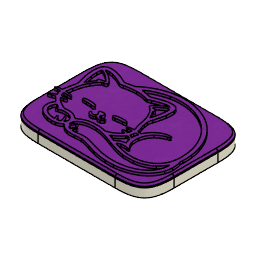
Sleeping Cat (Autodesk Fusion 360 design; units mm, degrees)
Autodesk Fusion 360 part; units mm, degrees
sketch "Imported SVG" plane through (0, 0, 0) normal (0, 0, 1) x (1, 0, 0)
  spline S0 degree 3 poles (44.1719, -83.1207) (37.6327, -82.7636) (28.995, -81.3586) (21.6671, -79.4603) knots 0 0 0 0 1 1 1 1
  spline S1 degree 3 poles (21.6671, -79.4603) (19.4843, -78.8948) (14.067, -77.2897) (9.6286, -75.8934) knots 0 0 0 0 1 1 1 1
  spline S2 degree 3 poles (9.6286, -75.8934) (0.5567, -73.0394) (-2.952, -72.1681) (-6.8676, -71.7971) knots 0 0 0 0 1 1 1 1
  spline S3 degree 3 poles (-6.8676, -71.7971) (-9.7124, -71.5276) (-14.5477, -71.7698) (-18.1526, -72.3625) knots 0 0 0 0 1 1 1 1
  spline S4 degree 3 poles (-18.1526, -72.3625) (-21.044, -72.8379) (-28.1463, -72.7506) (-30.562, -72.2099) knots 0 0 0 0 1 1 1 1
  spline S5 degree 3 poles (-30.562, -72.2099) (-33.3375, -71.5887) (-35.9478, -70.638) (-37.6802, -69.6171) knots 0 0 0 0 1 1 1 1
  spline S6 degree 3 poles (-37.6802, -69.6171) (-39.1993, -68.722) (-42.056, -66.0985) (-42.8145, -64.902) knots 0 0 0 0 1 1 1 1
  spline S7 degree 3 poles (-42.8145, -64.902) (-43.2338, -64.2406) (-43.2338, -64.2406) (-43.9885, -64.9292) knots 0 0 0 0 1 1 1 1
  spline S8 degree 3 poles (-43.9885, -64.9292) (-46.1715, -66.921) (-49.1149, -68.3543) (-53.2379, -69.4332) knots 0 0 0 0 1 1 1 1
  spline S9 degree 3 poles (-53.2379, -69.4332) (-55.2617, -69.9628) (-56.2025, -70.0467) (-59.9568, -70.0326) knots 0 0 0 0 1 1 1 1
  spline S10 degree 3 poles (-59.9568, -70.0326) (-63.7018, -70.0185) (-64.7913, -69.9128) (-67.6205, -69.2894) knots 0 0 0 0 1 1 1 1
  spline S11 degree 3 poles (-67.6205, -69.2894) (-75.9739, -67.4486) (-82.0673, -63.6492) (-85.307, -58.2616) knots 0 0 0 0 1 1 1 1
  spline S12 degree 3 poles (-85.307, -58.2616) (-85.6218, -57.738) (-86.2028, -56.4878) (-86.5979, -55.4834) knots 0 0 0 0 1 1 1 1
  spline S13 degree 3 poles (-86.5979, -55.4834) (-87.2545, -53.8147) (-87.3163, -53.3493) (-87.3142, -50.0854) knots 0 0 0 0 1 1 1 1
  spline S14 degree 3 poles (-87.3142, -50.0854) (-87.3121, -46.83) (-87.2471, -46.342) (-86.5803, -44.5775) knots 0 0 0 0 1 1 1 1
  spline S15 degree 3 poles (-86.5803, -44.5775) (-85.9476, -42.9035) (-84.7731, -40.6976) (-83.7154, -39.1965) knots 0 0 0 0 1 1 1 1
  spline S16 degree 3 poles (-83.7154, -39.1965) (-83.4549, -38.8267) (-83.6508, -38.5397) (-84.9772, -37.3485) knots 0 0 0 0 1 1 1 1
  spline S17 degree 3 poles (-84.9772, -37.3485) (-86.9937, -35.5374) (-88.0353, -34.4909) (-89.9901, -32.3117) knots 0 0 0 0 1 1 1 1
  spline S18 degree 3 poles (-89.9901, -32.3117) (-91.5745, -30.5454) (-91.5745, -30.5454) (-96.4559, -32.3963) knots 0 0 0 0 1 1 1 1
  spline S19 degree 3 poles (-96.4559, -32.3963) (-100.5126, -33.9346) (-101.4401, -34.2004) (-101.946, -33.9699) knots 0 0 0 0 1 1 1 1
  spline S20 degree 3 poles (-101.946, -33.9699) (-102.6861, -33.6327) (-102.7356, -32.8037) (-102.0562, -32.1243) knots 0 0 0 0 1 1 1 1
  spline S21 degree 3 poles (-102.0562, -32.1243) (-101.3048, -31.373) (-98.7657, -29.9625) (-95.8079, -28.6533) knots 0 0 0 0 1 1 1 1
  spline S22 degree 3 poles (-95.8079, -28.6533) (-94.3526, -28.0093) (-93.1244, -27.4603) (-93.0784, -27.4334) knots 0 0 0 0 1 1 1 1
  spline S23 degree 3 poles (-93.0784, -27.4334) (-93.0324, -27.4064) (-93.3604, -26.525) (-93.8074, -25.4747) knots 0 0 0 0 1 1 1 1
  spline S24 degree 3 poles (-93.8074, -25.4747) (-94.6338, -23.5327) (-95.411, -20.6554) (-95.411, -19.5379) knots 0 0 0 0 1 1 1 1
  spline S25 degree 3 poles (-95.411, -19.5379) (-95.411, -19.1987) (-95.5598, -18.8682) (-95.7417, -18.8034) knots 0 0 0 0 1 1 1 1
  spline S26 degree 3 poles (-95.7417, -18.8034) (-95.9236, -18.7386) (-97.998, -18.7963) (-100.3516, -18.9316) knots 0 0 0 0 1 1 1 1
  spline S27 degree 3 poles (-100.3516, -18.9316) (-105.0411, -19.2011) (-106.0471, -19.02) (-106.2103, -17.8766) knots 0 0 0 0 1 1 1 1
  spline S28 degree 3 poles (-106.2103, -17.8766) (-106.3839, -16.6604) (-104.273, -15.967) (-98.7253, -15.4178) knots 0 0 0 0 1 1 1 1
  spline S29 degree 3 poles (-98.7253, -15.4178) (-97.1284, -15.2597) (-95.8104, -15.1073) (-95.7963, -15.0792) knots 0 0 0 0 1 1 1 1
  spline S30 degree 3 poles (-95.7963, -15.0792) (-95.7821, -15.0511) (-95.6257, -13.6589) (-95.4487, -11.9854) knots 0 0 0 0 1 1 1 1
  spline S31 degree 3 poles (-95.4487, -11.9854) (-95.2716, -10.3119) (-94.7182, -7.2163) (-94.2189, -5.1062) knots 0 0 0 0 1 1 1 1
  spline S32 degree 3 poles (-94.2189, -5.1062) (-93.7196, -2.9962) (-92.9464, 0.5526) (-92.5007, 2.7798) knots 0 0 0 0 1 1 1 1
  spline S33 degree 3 poles (-92.5007, 2.7798) (-91.5958, 7.3017) (-91.4237, 5.8765) (-94.0568, 15.6636) knots 0 0 0 0 1 1 1 1
  spline S34 degree 3 poles (-94.0568, 15.6636) (-94.4874, 17.2643) (-95.1952, 20.3599) (-95.6295, 22.5427) knots 0 0 0 0 1 1 1 1
  spline S35 degree 3 poles (-95.6295, 22.5427) (-97.4372, 31.6271) (-98.0013, 37.4542) (-97.5381, 42.2569) knots 0 0 0 0 1 1 1 1
  spline S36 degree 3 poles (-97.5381, 42.2569) (-96.6603, 51.359) (-94.0135, 55.105) (-87.5048, 56.4575) knots 0 0 0 0 1 1 1 1
  spline S37 degree 3 poles (-87.5048, 56.4575) (-81.1549, 57.7769) (-69.2652, 54.9101) (-57.1426, 49.1368) knots 0 0 0 0 1 1 1 1
  spline S38 degree 3 poles (-57.1426, 49.1368) (-53.1378, 47.2295) (-53.1378, 47.2295) (-48.2791, 48.4514) knots 0 0 0 0 1 1 1 1
  spline S39 degree 3 poles (-48.2791, 48.4514) (-45.6068, 49.1235) (-42.2762, 49.8288) (-40.8778, 50.0188) knots 0 0 0 0 1 1 1 1
  spline S40 degree 3 poles (-40.8778, 50.0188) (-38.3352, 50.3643) (-38.3352, 50.3643) (-36.1153, 52.2914) knots 0 0 0 0 1 1 1 1
  spline S41 degree 3 poles (-36.1153, 52.2914) (-29.682, 57.8762) (-22.2779, 62.5427) (-14.0516, 66.1972) knots 0 0 0 0 1 1 1 1
  spline S42 degree 3 poles (-14.0516, 66.1972) (-5.5262, 69.9846) (3.8871, 72.5528) (13.2439, 73.6442) knots 0 0 0 0 1 1 1 1
  spline S43 degree 3 poles (13.2439, 73.6442) (18.3627, 74.2413) (27.6961, 74.2377) (32.5805, 73.6368) knots 0 0 0 0 1 1 1 1
  spline S44 degree 3 poles (32.5805, 73.6368) (51.3464, 71.328) (68.3594, 63.9806) (81.7612, 52.397) knots 0 0 0 0 1 1 1 1
  spline S45 degree 3 poles (81.7612, 52.397) (93.211, 42.5006) (101.58, 29.8071) (106.4162, 15.0021) knots 0 0 0 0 1 1 1 1
  spline S46 degree 3 poles (106.4162, 15.0021) (108.8797, 7.4607) (109.4869, 4.8611) (110.4334, -2.1958) knots 0 0 0 0 1 1 1 1
  spline S47 degree 3 poles (110.4334, -2.1958) (111.1822, -7.7792) (111.3768, -13.2405) (110.9863, -17.7108) knots 0 0 0 0 1 1 1 1
  spline S48 degree 3 poles (110.9863, -17.7108) (110.6856, -21.1527) (110.6986, -21.4838) (111.1978, -23.0979) knots 0 0 0 0 1 1 1 1
  spline S49 degree 3 poles (111.1978, -23.0979) (112.7036, -27.9673) (113.1723, -31.5404) (113.0055, -36.8779) knots 0 0 0 0 1 1 1 1
  spline S50 degree 3 poles (113.0055, -36.8779) (112.8526, -41.772) (112.3877, -44.5762) (111.0572, -48.6302) knots 0 0 0 0 1 1 1 1
  spline S51 degree 3 poles (111.0572, -48.6302) (104.9608, -67.2056) (84.7258, -80.447) (58.7088, -82.8859) knots 0 0 0 0 1 1 1 1
  spline S52 degree 3 poles (58.7088, -82.8859) (54.8482, -83.2478) (48.4048, -83.3519) (44.1719, -83.1207) knots 0 0 0 0 1 1 1 1
  spline S53 degree 3 poles (59.6349, -76.2813) (73.1592, -74.7946) (83.8175, -70.8695) (92.7216, -64.0966) knots 0 0 0 0 1 1 1 1
  spline S54 degree 3 poles (92.7216, -64.0966) (95.3009, -62.1347) (99.2539, -57.9512) (100.9411, -55.3979) knots 0 0 0 0 1 1 1 1
  spline S55 degree 3 poles (100.9411, -55.3979) (104.5866, -49.8809) (106.8783, -42.5825) (106.68, -37.1208) knots 0 0 0 0 1 1 1 1
  spline S56 degree 3 poles (106.68, -37.1208) (106.5984, -34.8718) (106.5984, -34.8718) (105.5401, -36.8541) knots 0 0 0 0 1 1 1 1
  spline S57 degree 3 poles (105.5401, -36.8541) (103.3997, -40.8631) (99.8697, -45.3493) (96.5442, -48.2865) knots 0 0 0 0 1 1 1 1
  spline S58 degree 3 poles (96.5442, -48.2865) (89.2838, -54.6995) (80.4809, -58.4766) (69.1599, -60.0365) knots 0 0 0 0 1 1 1 1
  spline S59 degree 3 poles (69.1599, -60.0365) (64.995, -60.6103) (55.3281, -60.6926) (51.6974, -60.1851) knots 0 0 0 0 1 1 1 1
  spline S60 degree 3 poles (51.6974, -60.1851) (42.5072, -58.9004) (35.3971, -56.9631) (23.1224, -52.3992) knots 0 0 0 0 1 1 1 1
  spline S61 degree 3 poles (23.1224, -52.3992) (7.5582, -46.6122) (-1.8118, -44.1125) (-10.4797, -43.4351) knots 0 0 0 0 1 1 1 1
  spline S62 degree 3 poles (-10.4797, -43.4351) (-23.6948, -42.4023) (-35.2995, -46.4923) (-38.7857, -53.4116) knots 0 0 0 0 1 1 1 1
  spline S63 degree 3 poles (-38.7857, -53.4116) (-39.7884, -55.4016) (-39.8384, -60.4041) (-38.8556, -60.4041) knots 0 0 0 0 1 1 1 1
  spline S64 degree 3 poles (-38.8556, -60.4041) (-38.7388, -60.4041) (-38.2981, -59.6118) (-37.8762, -58.6433) knots 0 0 0 0 1 1 1 1
  spline S65 degree 3 poles (-37.8762, -58.6433) (-36.5382, -55.572) (-33.1377, -52.733) (-31.534, -53.3484) knots 0 0 0 0 1 1 1 1
  spline S66 degree 3 poles (-31.534, -53.3484) (-30.8188, -53.6229) (-31.0673, -54.2427) (-32.5652, -55.9214) knots 0 0 0 0 1 1 1 1
  spline S67 degree 3 poles (-32.5652, -55.9214) (-34.5051, -58.0955) (-35.4015, -60.035) (-35.5543, -62.3885) knots 0 0 0 0 1 1 1 1
  spline S68 degree 3 poles (-35.5543, -62.3885) (-35.6564, -63.9611) (-35.6002, -64.3037) (-35.1818, -64.6592) knots 0 0 0 0 1 1 1 1
  spline S69 degree 3 poles (-35.1818, -64.6592) (-34.6213, -65.1355) (-32.1243, -66.225) (-31.5933, -66.225) knots 0 0 0 0 1 1 1 1
  spline S70 degree 3 poles (-31.5933, -66.225) (-31.3998, -66.225) (-31.0343, -65.6418) (-30.7812, -64.9291) knots 0 0 0 0 1 1 1 1
  spline S71 degree 3 poles (-30.7812, -64.9291) (-29.807, -62.1862) (-27.3938, -59.6388) (-25.7511, -59.6192) knots 0 0 0 0 1 1 1 1
  spline S72 degree 3 poles (-25.7511, -59.6192) (-24.6173, -59.6056) (-24.6328, -60.2158) (-25.8056, -61.7648) knots 0 0 0 0 1 1 1 1
  spline S73 degree 3 poles (-25.8056, -61.7648) (-26.9421, -63.266) (-27.6777, -65.0368) (-27.6777, -66.2721) knots 0 0 0 0 1 1 1 1
  spline S74 degree 3 poles (-27.6777, -66.2721) (-27.6777, -66.9827) (-27.617, -67.02) (-26.4209, -67.0453) knots 0 0 0 0 1 1 1 1
  spline S75 degree 3 poles (-26.4209, -67.0453) (-24.3172, -67.0897) (-20.4251, -66.9827) (-20.2518, -66.8756) knots 0 0 0 0 1 1 1 1
  spline S76 degree 3 poles (-20.2518, -66.8756) (-20.1103, -66.7881) (-14.6329, -66.0458) (-10.5986, -65.5674) knots 0 0 0 0 1 1 1 1
  spline S77 degree 3 poles (-10.5986, -65.5674) (-8.5699, -65.3268) (-3.2912, -65.84) (-0.0019, -66.5975) knots 0 0 0 0 1 1 1 1
  spline S78 degree 3 poles (-0.0019, -66.5975) (3.1146, -67.3153) (5.2671, -67.9321) (15.1684, -70.9449) knots 0 0 0 0 1 1 1 1
  spline S79 degree 3 poles (15.1684, -70.9449) (26.3524, -74.3481) (32.8284, -75.6052) (44.5536, -76.6492) knots 0 0 0 0 1 1 1 1
  spline S80 degree 3 poles (44.5536, -76.6492) (46.5618, -76.828) (56.9717, -76.574) (59.6349, -76.2813) knots 0 0 0 0 1 1 1 1
  spline S81 degree 3 poles (-60.311, -63.2584) (-60.4008, -62.5) (-60.8841, -61.0559) (-61.3848, -60.0494) knots 0 0 0 0 1 1 1 1
  spline S82 degree 3 poles (-61.3848, -60.0494) (-62.347, -58.1155) (-62.3668, -57.4937) (-61.4662, -57.4937) knots 0 0 0 0 1 1 1 1
  spline S83 degree 3 poles (-61.4662, -57.4937) (-59.9519, -57.4937) (-57.7892, -60.1153) (-57.1235, -62.7578) knots 0 0 0 0 1 1 1 1
  spline S84 degree 3 poles (-57.1235, -62.7578) (-56.6476, -64.6472) (-56.6458, -64.6477) (-53.5746, -63.819) knots 0 0 0 0 1 1 1 1
  spline S85 degree 3 poles (-53.5746, -63.819) (-51.5221, -63.2652) (-51.5221, -63.2652) (-51.3465, -61.8599) knots 0 0 0 0 1 1 1 1
  spline S86 degree 3 poles (-51.3465, -61.8599) (-51.0498, -59.4857) (-51.7827, -57.1192) (-53.6657, -54.3703) knots 0 0 0 0 1 1 1 1
  spline S87 degree 3 poles (-53.6657, -54.3703) (-54.5053, -53.1447) (-54.4826, -52.4666) (-53.602, -52.4666) knots 0 0 0 0 1 1 1 1
  spline S88 degree 3 poles (-53.602, -52.4666) (-51.5314, -52.4666) (-48.4862, -56.3441) (-48.1335, -59.4298) knots 0 0 0 0 1 1 1 1
  spline S89 degree 3 poles (-48.1335, -59.4298) (-47.9172, -61.3222) (-47.8561, -61.3697) (-46.8691, -60.413) knots 0 0 0 0 1 1 1 1
  spline S90 degree 3 poles (-46.8691, -60.413) (-42.5188, -56.1965) (-45.7992, -49.1698) (-53.2099, -46.8305) knots 0 0 0 0 1 1 1 1
  spline S91 degree 3 poles (-53.2099, -46.8305) (-58.3274, -45.2152) (-65.3333, -45.7312) (-70.4631, -48.1013) knots 0 0 0 0 1 1 1 1
  spline S92 degree 3 poles (-70.4631, -48.1013) (-72.5845, -49.0814) (-73.4099, -49.2264) (-73.9268, -48.7095) knots 0 0 0 0 1 1 1 1
  spline S93 degree 3 poles (-73.9268, -48.7095) (-74.4426, -48.1937) (-74.2989, -47.5783) (-73.3355, -46.1777) knots 0 0 0 0 1 1 1 1
  spline S94 degree 3 poles (-73.3355, -46.1777) (-72.4266, -44.8565) (-72.4266, -44.8565) (-75.3327, -43.3465) knots 0 0 0 0 1 1 1 1
  spline S95 degree 3 poles (-75.3327, -43.3465) (-76.9311, -42.516) (-78.3907, -41.8948) (-78.5763, -41.9661) knots 0 0 0 0 1 1 1 1
  spline S96 degree 3 poles (-78.5763, -41.9661) (-79.0603, -42.1518) (-80.8613, -45.6818) (-81.2862, -47.2775) knots 0 0 0 0 1 1 1 1
  spline S97 degree 3 poles (-81.2862, -47.2775) (-81.7686, -49.0894) (-81.7492, -52.3579) (-81.2473, -53.8086) knots 0 0 0 0 1 1 1 1
  spline S98 degree 3 poles (-81.2473, -53.8086) (-79.2284, -59.6441) (-70.8704, -64.1056) (-61.0444, -64.593) knots 0 0 0 0 1 1 1 1
  spline S99 degree 3 poles (-61.0444, -64.593) (-60.1477, -64.6375) (-60.1477, -64.6375) (-60.311, -63.2584) knots 0 0 0 0 1 1 1 1
  spline S100 degree 3 poles (66.9109, -55.1086) (75.3792, -54.1692) (82.5148, -51.7376) (88.7632, -47.662) knots 0 0 0 0 1 1 1 1
  spline S101 degree 3 poles (88.7632, -47.662) (92.3319, -45.3343) (96.8631, -40.7042) (98.8203, -37.3854) knots 0 0 0 0 1 1 1 1
  spline S102 degree 3 poles (98.8203, -37.3854) (103.0096, -30.2819) (104.614, -23.7663) (104.614, -13.8566) knots 0 0 0 0 1 1 1 1
  spline S103 degree 3 poles (104.614, -13.8566) (104.614, 5.351) (98.4698, 23.0203) (86.6665, 37.7563) knots 0 0 0 0 1 1 1 1
  spline S104 degree 3 poles (86.6665, 37.7563) (79.8375, 46.2821) (70.6136, 53.5105) (59.6349, 58.94) knots 0 0 0 0 1 1 1 1
  spline S105 degree 3 poles (59.6349, 58.94) (43.114, 67.1104) (24.0063, 69.5487) (5.9352, 65.7925) knots 0 0 0 0 1 1 1 1
  spline S106 degree 3 poles (5.9352, 65.7925) (-5.1547, 63.4874) (-18.1932, 57.8998) (-25.3878, 52.3691) knots 0 0 0 0 1 1 1 1
  spline S107 degree 3 poles (-25.3878, 52.3691) (-27.0664, 51.0788) (-27.0408, 50.7324) (-25.2663, 50.7249) knots 0 0 0 0 1 1 1 1
  spline S108 degree 3 poles (-25.2663, 50.7249) (-24.065, 50.7198) (-16.1305, 49.2885) (-14.1839, 48.7256) knots 0 0 0 0 1 1 1 1
  spline S109 degree 3 poles (-14.1839, 48.7256) (-11.2604, 47.8804) (-10.0532, 47.9214) (-7.5668, 48.9503) knots 0 0 0 0 1 1 1 1
  spline S110 degree 3 poles (-7.5668, 48.9503) (-6.3313, 49.4616) (-3.8688, 50.479) (-2.0947, 51.2112) knots 0 0 0 0 1 1 1 1
  spline S111 degree 3 poles (-2.0947, 51.2112) (1.6451, 52.7547) (6.6116, 54.3264) (11.103, 55.3877) knots 0 0 0 0 1 1 1 1
  spline S112 degree 3 poles (11.103, 55.3877) (13.8907, 56.0464) (14.7681, 56.1339) (18.6245, 56.1376) knots 0 0 0 0 1 1 1 1
  spline S113 degree 3 poles (18.6245, 56.1376) (22.0499, 56.1409) (23.2975, 56.043) (24.4178, 55.6831) knots 0 0 0 0 1 1 1 1
  spline S114 degree 3 poles (24.4178, 55.6831) (28.2868, 54.44) (30.3716, 51.8075) (31.0832, 47.2666) knots 0 0 0 0 1 1 1 1
  spline S115 degree 3 poles (31.0832, 47.2666) (31.4668, 44.8189) (31.2408, 37.4252) (30.6915, 34.449) knots 0 0 0 0 1 1 1 1
  spline S116 degree 3 poles (30.6915, 34.449) (29.3351, 27.1004) (28.1631, 22.3575) (26.1477, 16.0605) knots 0 0 0 0 1 1 1 1
  spline S117 degree 3 poles (26.1477, 16.0605) (24.2681, 10.188) (24.3531, 10.686) (24.821, 8.2876) knots 0 0 0 0 1 1 1 1
  spline S118 degree 3 poles (24.821, 8.2876) (25.0515, 7.1056) (25.4887, 4.4158) (25.7925, 2.3102) knots 0 0 0 0 1 1 1 1
  spline S119 degree 3 poles (25.7925, 2.3102) (26.2523, -0.8765) (26.5352, -1.9637) (27.4802, -4.1762) knots 0 0 0 0 1 1 1 1
  spline S120 degree 3 poles (27.4802, -4.1762) (28.9055, -7.5131) (29.4228, -9.0202) (29.8883, -11.1916) knots 0 0 0 0 1 1 1 1
  spline S121 degree 3 poles (29.8883, -11.1916) (30.091, -12.1375) (30.259, -12.9827) (30.2615, -13.0699) knots 0 0 0 0 1 1 1 1
  spline S122 degree 3 poles (30.2615, -13.0699) (30.2642, -13.157) (31.4297, -13.2992) (32.8519, -13.3859) knots 0 0 0 0 1 1 1 1
  spline S123 degree 3 poles (32.8519, -13.3859) (34.2741, -13.4725) (35.6339, -13.6187) (35.8737, -13.7107) knots 0 0 0 0 1 1 1 1
  spline S124 degree 3 poles (35.8737, -13.7107) (36.2182, -13.8429) (36.5584, -13.3605) (37.4959, -11.4103) knots 0 0 0 0 1 1 1 1
  spline S125 degree 3 poles (37.4959, -11.4103) (40.5115, -5.1373) (45.9211, 0.448) (52.5205, 4.1023) knots 0 0 0 0 1 1 1 1
  spline S126 degree 3 poles (52.5205, 4.1023) (56.4485, 6.2774) (63.9968, 8.2004) (66.2379, 7.5969) knots 0 0 0 0 1 1 1 1
  spline S127 degree 3 poles (66.2379, 7.5969) (67.8756, 7.1559) (68.2609, 5.9132) (66.963, 5.2582) knots 0 0 0 0 1 1 1 1
  spline S128 degree 3 poles (66.963, 5.2582) (66.6433, 5.0968) (65.0944, 4.4824) (63.5211, 3.8928) knots 0 0 0 0 1 1 1 1
  spline S129 degree 3 poles (63.5211, 3.8928) (57.362, 1.5846) (53.089, -1.0306) (49.3287, -4.7934) knots 0 0 0 0 1 1 1 1
  spline S130 degree 3 poles (49.3287, -4.7934) (44.5974, -9.5279) (41.7411, -15.1078) (40.4331, -22.1718) knots 0 0 0 0 1 1 1 1
  spline S131 degree 3 poles (40.4331, -22.1718) (39.8445, -25.3509) (40.0269, -30.5204) (40.8394, -33.6812) knots 0 0 0 0 1 1 1 1
  spline S132 degree 3 poles (40.8394, -33.6812) (41.8295, -37.5332) (44.0548, -41.3179) (46.515, -43.3338) knots 0 0 0 0 1 1 1 1
  spline S133 degree 3 poles (46.515, -43.3338) (47.8461, -44.4245) (48.1562, -45.0531) (47.7436, -45.8241) knots 0 0 0 0 1 1 1 1
  spline S134 degree 3 poles (47.7436, -45.8241) (47.2915, -46.6687) (46.5064, -46.73) (44.4747, -46.0792) knots 0 0 0 0 1 1 1 1
  spline S135 degree 3 poles (44.4747, -46.0792) (41.9167, -45.2599) (36.4787, -45.1891) (34.2349, -45.946) knots 0 0 0 0 1 1 1 1
  spline S136 degree 3 poles (34.2349, -45.946) (32.6269, -46.4885) (29.2078, -48.3928) (29.2078, -48.746) knots 0 0 0 0 1 1 1 1
  spline S137 degree 3 poles (29.2078, -48.746) (29.2078, -49.0172) (29.3883, -49.0891) (32.912, -50.2209) knots 0 0 0 0 1 1 1 1
  spline S138 degree 3 poles (32.912, -50.2209) (41.6344, -53.0228) (46.4035, -54.147) (53.5495, -55.0858) knots 0 0 0 0 1 1 1 1
  spline S139 degree 3 poles (53.5495, -55.0858) (55.9955, -55.4071) (64.0948, -55.4209) (66.9109, -55.1086) knots 0 0 0 0 1 1 1 1
  spline S140 degree 3 poles (-39.2437, -45.4444) (-36.2715, -42.9976) (-31.4062, -40.6886) (-26.7516, -39.516) knots 0 0 0 0 1 1 1 1
  spline S141 degree 3 poles (-26.7516, -39.516) (-18.8801, -37.533) (-8.5354, -37.648) (-0.4924, -39.8081) knots 0 0 0 0 1 1 1 1
  spline S142 degree 3 poles (-0.4924, -39.8081) (1.4251, -40.323) (1.4251, -40.323) (3.8155, -39.3666) knots 0 0 0 0 1 1 1 1
  spline S143 degree 3 poles (3.8155, -39.3666) (8.8608, -37.3481) (12.3833, -35.3802) (15.5817, -32.7935) knots 0 0 0 0 1 1 1 1
  spline S144 degree 3 poles (15.5817, -32.7935) (17.8654, -30.9465) (21.0057, -27.5683) (21.0057, -26.9586) knots 0 0 0 0 1 1 1 1
  spline S145 degree 3 poles (21.0057, -26.9586) (21.0057, -26.7983) (19.7083, -26.3304) (18.1227, -25.9188) knots 0 0 0 0 1 1 1 1
  spline S146 degree 3 poles (18.1227, -25.9188) (14.8583, -25.0715) (14.1265, -24.672) (14.1265, -23.7378) knots 0 0 0 0 1 1 1 1
  spline S147 degree 3 poles (14.1265, -23.7378) (14.1265, -22.5286) (16.3638, -22.2306) (19.8151, -22.9801) knots 0 0 0 0 1 1 1 1
  spline S148 degree 3 poles (19.8151, -22.9801) (20.8337, -23.2014) (21.974, -23.4482) (22.3491, -23.5286) knots 0 0 0 0 1 1 1 1
  spline S149 degree 3 poles (22.3491, -23.5286) (22.9979, -23.6678) (23.0593, -23.5799) (23.6124, -21.7166) knots 0 0 0 0 1 1 1 1
  spline S150 degree 3 poles (23.6124, -21.7166) (23.9322, -20.6395) (24.2692, -19.1213) (24.3614, -18.3428) knots 0 0 0 0 1 1 1 1
  spline S151 degree 3 poles (24.3614, -18.3428) (24.529, -16.9274) (24.529, -16.9274) (21.9075, -17.0996) knots 0 0 0 0 1 1 1 1
  spline S152 degree 3 poles (21.9075, -17.0996) (20.4656, -17.1943) (18.3929, -17.3469) (17.3015, -17.4387) knots 0 0 0 0 1 1 1 1
  spline S153 degree 3 poles (17.3015, -17.4387) (15.5803, -17.5834) (15.2337, -17.5377) (14.6882, -17.0941) knots 0 0 0 0 1 1 1 1
  spline S154 degree 3 poles (14.6882, -17.0941) (13.8319, -16.3979) (14.1225, -15.5899) (15.4152, -15.0727) knots 0 0 0 0 1 1 1 1
  spline S155 degree 3 poles (15.4152, -15.0727) (16.789, -14.523) (20.0865, -13.8637) (22.4697, -13.6622) knots 0 0 0 0 1 1 1 1
  spline S156 degree 3 poles (22.4697, -13.6622) (23.5563, -13.5704) (24.4453, -13.3995) (24.4453, -13.2825) knots 0 0 0 0 1 1 1 1
  spline S157 degree 3 poles (24.4453, -13.2825) (24.4453, -12.4787) (23.6582, -9.7532) (22.5748, -6.8059) knots 0 0 0 0 1 1 1 1
  spline S158 degree 3 poles (22.5748, -6.8059) (21.1724, -2.9903) (20.7374, -1.3038) (20.089, 2.8313) knots 0 0 0 0 1 1 1 1
  spline S159 degree 3 poles (20.089, 2.8313) (18.8589, 10.6764) (16.863, 16.5202) (13.5059, 22.1056) knots 0 0 0 0 1 1 1 1
  spline S160 degree 3 poles (13.5059, 22.1056) (10.2542, 27.5157) (7.6384, 30.5938) (5.4824, 31.5473) knots 0 0 0 0 1 1 1 1
  spline S161 degree 3 poles (5.4824, 31.5473) (1.7067, 33.2171) (1.7839, 35.2706) (5.7707, 39.2128) knots 0 0 0 0 1 1 1 1
  spline S162 degree 3 poles (5.7707, 39.2128) (9.5962, 42.9955) (16.0602, 47.3872) (20.0222, 48.8956) knots 0 0 0 0 1 1 1 1
  spline S163 degree 3 poles (20.0222, 48.8956) (20.8638, 49.2159) (21.5093, 49.6069) (21.4568, 49.7644) knots 0 0 0 0 1 1 1 1
  spline S164 degree 3 poles (21.4568, 49.7644) (21.2645, 50.3413) (19.0711, 50.5363) (16.2432, 50.228) knots 0 0 0 0 1 1 1 1
  spline S165 degree 3 poles (16.2432, 50.228) (10.9478, 49.6507) (3.508, 47.2744) (-3.8764, 43.8018) knots 0 0 0 0 1 1 1 1
  spline S166 degree 3 poles (-3.8764, 43.8018) (-6.0778, 42.7666) (-8.3749, 41.8655) (-8.9809, 41.7994) knots 0 0 0 0 1 1 1 1
  spline S167 degree 3 poles (-8.9809, 41.7994) (-9.6841, 41.7228) (-10.9924, 41.9288) (-12.5964, 42.3689) knots 0 0 0 0 1 1 1 1
  spline S168 degree 3 poles (-12.5964, 42.3689) (-18.8446, 44.0833) (-23.2549, 44.6822) (-29.662, 44.6864) knots 0 0 0 0 1 1 1 1
  spline S169 degree 3 poles (-29.662, 44.6864) (-35.9239, 44.6906) (-44.1564, 43.584) (-49.638, 42.0013) knots 0 0 0 0 1 1 1 1
  spline S170 degree 3 poles (-49.638, 42.0013) (-53.6753, 40.8356) (-54.0853, 40.8802) (-58.3381, 42.9464) knots 0 0 0 0 1 1 1 1
  spline S171 degree 3 poles (-58.3381, 42.9464) (-64.8679, 46.119) (-70.0753, 48.122) (-75.2325, 49.4448) knots 0 0 0 0 1 1 1 1
  spline S172 degree 3 poles (-75.2325, 49.4448) (-78.187, 50.2026) (-79.0407, 50.3119) (-82.0495, 50.3175) knots 0 0 0 0 1 1 1 1
  spline S173 degree 3 poles (-82.0495, 50.3175) (-85.2976, 50.3236) (-87.2089, 49.985) (-87.2089, 49.4035) knots 0 0 0 0 1 1 1 1
  spline S174 degree 3 poles (-87.2089, 49.4035) (-87.2089, 49.2964) (-86.1563, 48.7724) (-84.8698, 48.2392) knots 0 0 0 0 1 1 1 1
  spline S175 degree 3 poles (-84.8698, 48.2392) (-79.9134, 46.1848) (-73.4744, 41.7938) (-69.3339, 37.6446) knots 0 0 0 0 1 1 1 1
  spline S176 degree 3 poles (-69.3339, 37.6446) (-66.7351, 35.0403) (-65.7776, 33.4502) (-65.7776, 31.7385) knots 0 0 0 0 1 1 1 1
  spline S177 degree 3 poles (-65.7776, 31.7385) (-65.7776, 29.9729) (-66.5587, 29.4404) (-69.7323, 29.0425) knots 0 0 0 0 1 1 1 1
  spline S178 degree 3 poles (-69.7323, 29.0425) (-71.03, 28.8798) (-72.2654, 28.555) (-72.7678, 28.2444) knots 0 0 0 0 1 1 1 1
  spline S179 degree 3 poles (-72.7678, 28.2444) (-74.4404, 27.2107) (-78.6948, 21.5955) (-81.2975, 16.9865) knots 0 0 0 0 1 1 1 1
  spline S180 degree 3 poles (-81.2975, 16.9865) (-84.7376, 10.8947) (-86.1306, 6.5198) (-88.2904, -4.9739) knots 0 0 0 0 1 1 1 1
  spline S181 degree 3 poles (-88.2904, -4.9739) (-89.5643, -11.7537) (-90.1102, -14.742) (-90.115, -14.9619) knots 0 0 0 0 1 1 1 1
  spline S182 degree 3 poles (-90.115, -14.9619) (-90.1174, -15.0711) (-89.5896, -15.1604) (-88.9422, -15.1604) knots 0 0 0 0 1 1 1 1
  spline S183 degree 3 poles (-88.9422, -15.1604) (-87.313, -15.1604) (-82.0795, -15.8765) (-80.3793, -16.3321) knots 0 0 0 0 1 1 1 1
  spline S184 degree 3 poles (-80.3793, -16.3321) (-79.6062, -16.5392) (-78.6835, -16.8989) (-78.3288, -17.1313) knots 0 0 0 0 1 1 1 1
  spline S185 degree 3 poles (-78.3288, -17.1313) (-77.574, -17.6258) (-77.4517, -18.792) (-78.1274, -19.0513) knots 0 0 0 0 1 1 1 1
  spline S186 degree 3 poles (-78.1274, -19.0513) (-78.3713, -19.1449) (-81.0204, -19.0943) (-84.0144, -18.9389) knots 0 0 0 0 1 1 1 1
  spline S187 degree 3 poles (-84.0144, -18.9389) (-87.0083, -18.7834) (-89.5365, -18.7035) (-89.6326, -18.7613) knots 0 0 0 0 1 1 1 1
  spline S188 degree 3 poles (-89.6326, -18.7613) (-89.9038, -18.9246) (-89.1407, -21.8772) (-88.3334, -23.7881) knots 0 0 0 0 1 1 1 1
  spline S189 degree 3 poles (-88.3334, -23.7881) (-87.4966, -25.7688) (-87.8995, -25.6863) (-83.2401, -24.83) knots 0 0 0 0 1 1 1 1
  spline S190 degree 3 poles (-83.2401, -24.83) (-80.2467, -24.2798) (-78.0316, -24.381) (-77.5119, -25.0917) knots 0 0 0 0 1 1 1 1
  spline S191 degree 3 poles (-77.5119, -25.0917) (-76.6783, -26.2318) (-77.347, -26.6716) (-81.4745, -27.6974) knots 0 0 0 0 1 1 1 1
  spline S192 degree 3 poles (-81.4745, -27.6974) (-83.4866, -28.1975) (-85.2128, -28.6865) (-85.3104, -28.7841) knots 0 0 0 0 1 1 1 1
  spline S193 degree 3 poles (-85.3104, -28.7841) (-85.6383, -29.112) (-80.7514, -33.558) (-78.213, -35.2411) knots 0 0 0 0 1 1 1 1
  spline S194 degree 3 poles (-78.213, -35.2411) (-75.4743, -37.0571) (-67.9126, -40.8684) (-66.1043, -41.3443) knots 0 0 0 0 1 1 1 1
  spline S195 degree 3 poles (-66.1043, -41.3443) (-65.2822, -41.5607) (-64.7073, -41.5629) (-63.9876, -41.3524) knots 0 0 0 0 1 1 1 1
  spline S196 degree 3 poles (-63.9876, -41.3524) (-63.4442, -41.1935) (-61.6303, -40.9992) (-59.9568, -40.9206) knots 0 0 0 0 1 1 1 1
  spline S197 degree 3 poles (-59.9568, -40.9206) (-56.3212, -40.7498) (-52.7148, -41.3582) (-49.5484, -42.6764) knots 0 0 0 0 1 1 1 1
  spline S198 degree 3 poles (-49.5484, -42.6764) (-47.5095, -43.5252) (-44.7643, -45.2163) (-43.9313, -46.1367) knots 0 0 0 0 1 1 1 1
  spline S199 degree 3 poles (-43.9313, -46.1367) (-43.5885, -46.5155) (-43.1164, -46.6458) (-42.0868, -46.6458) knots 0 0 0 0 1 1 1 1
  spline S200 degree 3 poles (-42.0868, -46.6458) (-40.8356, -46.6458) (-40.5632, -46.5308) (-39.2437, -45.4444) knots 0 0 0 0 1 1 1 1
  spline S201 degree 3 poles (-35.5835, -29.1588) (-39.0508, -28.1002) (-41.4441, -24.2206) (-39.1644, -23.3539) knots 0 0 0 0 1 1 1 1
  spline S202 degree 3 poles (-39.1644, -23.3539) (-38.3004, -23.0254) (-37.4523, -23.4009) (-36.8058, -24.3983) knots 0 0 0 0 1 1 1 1
  spline S203 degree 3 poles (-36.8058, -24.3983) (-35.3391, -26.6607) (-32.0108, -26.5194) (-29.9459, -24.107) knots 0 0 0 0 1 1 1 1
  spline S204 degree 3 poles (-29.9459, -24.107) (-28.4931, -22.4098) (-28.5397, -21.92) (-30.3361, -19.9996) knots 0 0 0 0 1 1 1 1
  spline S205 degree 3 poles (-30.3361, -19.9996) (-32.289, -17.9119) (-32.6366, -16.6953) (-31.532, -15.8145) knots 0 0 0 0 1 1 1 1
  spline S206 degree 3 poles (-31.532, -15.8145) (-29.6661, -14.3267) (-24.2581, -14.367) (-22.5849, -15.8813) knots 0 0 0 0 1 1 1 1
  spline S207 degree 3 poles (-22.5849, -15.8813) (-21.6636, -16.7151) (-22.3061, -18.6897) (-24.17, -20.7529) knots 0 0 0 0 1 1 1 1
  spline S208 degree 3 poles (-24.17, -20.7529) (-25.1374, -21.8237) (-25.1374, -21.8237) (-24.4971, -23.0305) knots 0 0 0 0 1 1 1 1
  spline S209 degree 3 poles (-24.4971, -23.0305) (-23.7977, -24.349) (-22.2701, -25.6109) (-21.0487, -25.8792) knots 0 0 0 0 1 1 1 1
  spline S210 degree 3 poles (-21.0487, -25.8792) (-19.8331, -26.1462) (-18.5821, -25.5725) (-17.2675, -24.1454) knots 0 0 0 0 1 1 1 1
  spline S211 degree 3 poles (-17.2675, -24.1454) (-16.0382, -22.8109) (-15.4039, -22.5714) (-14.6683, -23.164) knots 0 0 0 0 1 1 1 1
  spline S212 degree 3 poles (-14.6683, -23.164) (-14.0009, -23.7018) (-13.9392, -24.276) (-14.4312, -25.372) knots 0 0 0 0 1 1 1 1
  spline S213 degree 3 poles (-14.4312, -25.372) (-15.1112, -26.8871) (-16.8054, -28.2908) (-18.5747, -28.8051) knots 0 0 0 0 1 1 1 1
  spline S214 degree 3 poles (-18.5747, -28.8051) (-21.2488, -29.5825) (-23.7247, -28.8632) (-25.7972, -26.7069) knots 0 0 0 0 1 1 1 1
  spline S215 degree 3 poles (-25.7972, -26.7069) (-26.6949, -25.7729) (-26.6949, -25.7729) (-27.7857, -26.8953) knots 0 0 0 0 1 1 1 1
  spline S216 degree 3 poles (-27.7857, -26.8953) (-28.3857, -27.5127) (-29.4479, -28.2943) (-30.1462, -28.6324) knots 0 0 0 0 1 1 1 1
  spline S217 degree 3 poles (-30.1462, -28.6324) (-31.5893, -29.331) (-34.1936, -29.5831) (-35.5835, -29.1588) knots 0 0 0 0 1 1 1 1
  spline S218 degree 3 poles (-48.8443, -13.6677) (-50.0812, -13.4622) (-53.9562, -13.208) (-57.4553, -13.1028) knots 0 0 0 0 1 1 1 1
  spline S219 degree 3 poles (-57.4553, -13.1028) (-62.8887, -12.9393) (-63.9219, -12.8429) (-64.5329, -12.4423) knots 0 0 0 0 1 1 1 1
  spline S220 degree 3 poles (-64.5329, -12.4423) (-65.3877, -11.8819) (-65.4718, -10.9466) (-64.728, -10.2735) knots 0 0 0 0 1 1 1 1
  spline S221 degree 3 poles (-64.728, -10.2735) (-62.7865, -8.5164) (-53.9533, -8.0641) (-47.2568, -9.3788) knots 0 0 0 0 1 1 1 1
  spline S222 degree 3 poles (-47.2568, -9.3788) (-44.5711, -9.9061) (-43.0235, -11.0155) (-43.0235, -12.4134) knots 0 0 0 0 1 1 1 1
  spline S223 degree 3 poles (-43.0235, -12.4134) (-43.0235, -14.1129) (-44.391, -14.4076) (-48.8443, -13.6677) knots 0 0 0 0 1 1 1 1
  spline S224 degree 3 poles (-13.0502, -12.9177) (-14.623, -12.2339) (-14.4667, -10.3527) (-12.77, -9.546) knots 0 0 0 0 1 1 1 1
  spline S225 degree 3 poles (-12.77, -9.546) (-8.715, -7.6179) (1.1061, -6.6965) (5.3886, -7.8424) knots 0 0 0 0 1 1 1 1
  spline S226 degree 3 poles (5.3886, -7.8424) (7.3925, -8.3785) (8.365, -9.1531) (8.2516, -10.1226) knots 0 0 0 0 1 1 1 1
  spline S227 degree 3 poles (8.2516, -10.1226) (8.1258, -11.1976) (7.0677, -11.4971) (2.5143, -11.7463) knots 0 0 0 0 1 1 1 1
  spline S228 degree 3 poles (2.5143, -11.7463) (-1.8955, -11.9876) (-4.9339, -12.3044) (-8.7599, -12.9219) knots 0 0 0 0 1 1 1 1
  spline S229 degree 3 poles (-8.7599, -12.9219) (-11.6492, -13.3882) (-11.9689, -13.3878) (-13.0502, -12.9177) knots 0 0 0 0 1 1 1 1
  spline S230 degree 3 poles (25.1971, -44.9761) (28.5331, -42.2608) (31.2046, -41.0068) (35.1378, -40.3103) knots 0 0 0 0 1 1 1 1
  spline S231 degree 3 poles (35.1378, -40.3103) (35.9983, -40.1579) (36.7388, -39.9967) (36.7834, -39.9521) knots 0 0 0 0 1 1 1 1
  spline S232 degree 3 poles (36.7834, -39.9521) (36.8281, -39.9074) (36.5169, -38.9755) (36.0919, -37.8811) knots 0 0 0 0 1 1 1 1
  spline S233 degree 3 poles (36.0919, -37.8811) (35.667, -36.7867) (35.0929, -34.7689) (34.8162, -33.3972) knots 0 0 0 0 1 1 1 1
  spline S234 degree 3 poles (34.8162, -33.3972) (34.3132, -30.9031) (34.3132, -30.9031) (33.1496, -30.4539) knots 0 0 0 0 1 1 1 1
  spline S235 degree 3 poles (33.1496, -30.4539) (30.5936, -29.4672) (27.5622, -28.3895) (27.3429, -28.3895) knots 0 0 0 0 1 1 1 1
  spline S236 degree 3 poles (27.3429, -28.3895) (27.2153, -28.3895) (26.6335, -29.0925) (26.05, -29.9517) knots 0 0 0 0 1 1 1 1
  spline S237 degree 3 poles (26.05, -29.9517) (23.4907, -33.7204) (18.7929, -37.9062) (13.8164, -40.8519) knots 0 0 0 0 1 1 1 1
  spline S238 degree 3 poles (13.8164, -40.8519) (12.5251, -41.6163) (11.5606, -42.3301) (11.6731, -42.4383) knots 0 0 0 0 1 1 1 1
  spline S239 degree 3 poles (11.6731, -42.4383) (11.7856, -42.5464) (13.3659, -43.1773) (15.1849, -43.8403) knots 0 0 0 0 1 1 1 1
  spline S240 degree 3 poles (15.1849, -43.8403) (17.0039, -44.5033) (19.3851, -45.3938) (20.4765, -45.8193) knots 0 0 0 0 1 1 1 1
  spline S241 degree 3 poles (20.4765, -45.8193) (21.5679, -46.2448) (22.615, -46.6048) (22.8034, -46.6193) knots 0 0 0 0 1 1 1 1
  spline S242 degree 3 poles (22.8034, -46.6193) (22.9917, -46.6339) (24.0689, -45.8944) (25.1971, -44.9761) knots 0 0 0 0 1 1 1 1
  spline S243 degree 3 poles (34.0956, -24.8838) (34.1954, -23.5377) (34.5057, -21.2866) (34.7851, -19.8813) knots 0 0 0 0 1 1 1 1
  spline S244 degree 3 poles (34.7851, -19.8813) (35.0645, -18.476) (35.2932, -17.2512) (35.2932, -17.1594) knots 0 0 0 0 1 1 1 1
  spline S245 degree 3 poles (35.2932, -17.1594) (35.2932, -17.0677) (34.1925, -17.0268) (32.8472, -17.0687) knots 0 0 0 0 1 1 1 1
  spline S246 degree 3 poles (32.8472, -17.0687) (30.4013, -17.1448) (30.4013, -17.1448) (29.9326, -19.9229) knots 0 0 0 0 1 1 1 1
  spline S247 degree 3 poles (29.9326, -19.9229) (29.6748, -21.4508) (29.2876, -23.2272) (29.072, -23.8704) knots 0 0 0 0 1 1 1 1
  spline S248 degree 3 poles (29.072, -23.8704) (28.8565, -24.5135) (28.7219, -25.0814) (28.7729, -25.1324) knots 0 0 0 0 1 1 1 1
  spline S249 degree 3 poles (28.7729, -25.1324) (28.8924, -25.2519) (33.5185, -27.2762) (33.7437, -27.3075) knots 0 0 0 0 1 1 1 1
  spline S250 degree 3 poles (33.7437, -27.3075) (33.8374, -27.3206) (33.9958, -26.2299) (34.0956, -24.8838) knots 0 0 0 0 1 1 1 1
  spline S251 degree 3 poles (-86.0421, 15.8486) (-84.6829, 18.7247) (-83.0131, 21.4711) (-80.7848, 24.4958) knots 0 0 0 0 1 1 1 1
  spline S252 degree 3 poles (-80.7848, 24.4958) (-79.3867, 26.3937) (-79.04, 27.0312) (-79.3122, 27.2038) knots 0 0 0 0 1 1 1 1
  spline S253 degree 3 poles (-79.3122, 27.2038) (-79.508, 27.3279) (-79.7605, 27.4313) (-79.8733, 27.4335) knots 0 0 0 0 1 1 1 1
  spline S254 degree 3 poles (-79.8733, 27.4335) (-79.986, 27.4356) (-80.2014, 27.7616) (-80.352, 28.1576) knots 0 0 0 0 1 1 1 1
  spline S255 degree 3 poles (-80.352, 28.1576) (-81.0891, 30.0962) (-79.1354, 31.07) (-71.4, 32.62) knots 0 0 0 0 1 1 1 1
  spline S256 degree 3 poles (-71.4, 32.62) (-71.0726, 32.6856) (-70.8047, 32.873) (-70.8047, 33.0364) knots 0 0 0 0 1 1 1 1
  spline S257 degree 3 poles (-70.8047, 33.0364) (-70.8047, 34.1654) (-77.1278, 39.7369) (-81.4272, 42.3964) knots 0 0 0 0 1 1 1 1
  spline S258 degree 3 poles (-81.4272, 42.3964) (-84.6283, 44.3766) (-89.049, 46.5276) (-89.7196, 46.4315) knots 0 0 0 0 1 1 1 1
  spline S259 degree 3 poles (-89.7196, 46.4315) (-90.0347, 46.3863) (-90.4673, 45.9238) (-90.7808, 45.2969) knots 0 0 0 0 1 1 1 1
  spline S260 degree 3 poles (-90.7808, 45.2969) (-91.2626, 44.3332) (-91.3093, 43.718) (-91.3027, 38.4177) knots 0 0 0 0 1 1 1 1
  spline S261 degree 3 poles (-91.3027, 38.4177) (-91.2967, 33.6409) (-91.1856, 31.9088) (-90.6832, 28.7605) knots 0 0 0 0 1 1 1 1
  spline S262 degree 3 poles (-90.6832, 28.7605) (-89.987, 24.3982) (-89.0686, 19.9632) (-88.122, 16.3924) knots 0 0 0 0 1 1 1 1
  spline S263 degree 3 poles (-88.122, 16.3924) (-87.7653, 15.047) (-87.4735, 13.8861) (-87.4735, 13.8127) knots 0 0 0 0 1 1 1 1
  spline S264 degree 3 poles (-87.4735, 13.8127) (-87.4735, 13.7393) (-87.3821, 13.6792) (-87.2704, 13.6792) knots 0 0 0 0 1 1 1 1
  spline S265 degree 3 poles (-87.2704, 13.6792) (-87.1587, 13.6792) (-86.6059, 14.6554) (-86.0421, 15.8486) knots 0 0 0 0 1 1 1 1
  spline S266 degree 3 poles (20.6999, 19.0539) (21.9411, 22.3712) (23.8002, 30.5203) (24.5698, 36.0164) knots 0 0 0 0 1 1 1 1
  spline S267 degree 3 poles (24.5698, 36.0164) (25.0653, 39.5554) (25.0989, 44.5049) (24.6338, 45.4292) knots 0 0 0 0 1 1 1 1
  spline S268 degree 3 poles (24.6338, 45.4292) (24.4047, 45.8844) (24.0431, 46.1159) (23.4738, 46.1716) knots 0 0 0 0 1 1 1 1
  spline S269 degree 3 poles (23.4738, 46.1716) (21.2727, 46.3869) (13.6269, 41.5278) (8.901, 36.9103) knots 0 0 0 0 1 1 1 1
  spline S270 degree 3 poles (8.901, 36.9103) (7.1267, 35.1767) (6.9035, 34.6619) (7.8427, 34.4692) knots 0 0 0 0 1 1 1 1
  spline S271 degree 3 poles (7.8427, 34.4692) (10.7224, 33.8782) (11.5179, 33.6907) (12.6713, 33.3314) knots 0 0 0 0 1 1 1 1
  spline S272 degree 3 poles (12.6713, 33.3314) (14.5916, 32.7332) (15.4494, 32.0562) (15.4494, 31.1387) knots 0 0 0 0 1 1 1 1
  spline S273 degree 3 poles (15.4494, 31.1387) (15.4494, 30.2806) (14.634, 29.5542) (13.6708, 29.5542) knots 0 0 0 0 1 1 1 1
  spline S274 degree 3 poles (13.6708, 29.5542) (13.3393, 29.5542) (13.0682, 29.4626) (13.0682, 29.3506) knots 0 0 0 0 1 1 1 1
  spline S275 degree 3 poles (13.0682, 29.3506) (13.0682, 29.2386) (13.6009, 28.4349) (14.2521, 27.5646) knots 0 0 0 0 1 1 1 1
  spline S276 degree 3 poles (14.2521, 27.5646) (15.6326, 25.7195) (18.3736, 20.968) (19.1882, 19.0078) knots 0 0 0 0 1 1 1 1
  spline S277 degree 3 poles (19.1882, 19.0078) (19.499, 18.2599) (19.8479, 17.6479) (19.9636, 17.6479) knots 0 0 0 0 1 1 1 1
  spline S278 degree 3 poles (19.9636, 17.6479) (20.0793, 17.6479) (20.4106, 18.2806) (20.6999, 19.0539) knots 0 0 0 0 1 1 1 1
  line L0 (119.968, -91.5939) -> (-110.6847, -91.5939)
  line L1 (-110.6847, -91.5939) -> (-110.6847, 82.8194)
  line L2 (-110.6847, 82.8194) -> (119.968, 82.8194)
  line L3 (119.968, 82.8194) -> (119.968, -91.5939)
  constraint horizontal L0
  constraint vertical L1
  constraint horizontal L2
  constraint vertical L3
extrude "Extrude1" add sketch "Imported SVG" against normal blind 5 contours S0 S1 S2 S3 S4 S5 S6 S7 S8 S9 S10 S11 S12 S13 S14 S15 S16 S17 S18 S19 S20 S21 S22 S23 S24 S25 S26 S27 S28 S29 S30 S31 S32 S33 S34 S35 S36 S37 S38 S39 S40 S41 S42 S43 S44 S45 S46 S47 S48 S49 S50 S51 S52 | S53 S54 S55 S56 S57 S58 S59 S60 S61 S62 S63 S64 S65 S66 S67 S68 S69 S70 S71 S72 S73 S74 S75 S76 S77 S78 S79 S80 | S81 S82 S83 S84 S85 S86 S87 S88 S89 S90 S91 S92 S93 S94 S95 S96 S97 S98 S99 | S100 S101 S102 S103 S104 S105 S106 S107 S108 S109 S110 S111 S112 S113 S114 S115 S116 S117 S118 S119 S120 S121 S122 S123 S124 S125 S126 S127 S128 S129 S130 S131 S132 S133 S134 S135 S136 S137 S138 S139 | S140 S141 S142 S143 S144 S145 S146 S147 S148 S149 S150 S151 S152 S153 S154 S155 S156 S157 S158 S159 S160 S161 S162 S163 S164 S165 S166 S167 S168 S169 S170 S171 S172 S173 S174 S175 S176 S177 S178 S179 S180 S181 S182 S183 S184 S185 S186 S187 S188 S189 S190 S191 S192 S193 S194 S195 S196 S197 S198 S199 S200 | S201 S202 S203 S204 S205 S206 S207 S208 S209 S210 S211 S212 S213 S214 S215 S216 S217 | S218 S219 S220 S221 S222 S223 | S224 S225 S226 S227 S228 S229 | S230 S231 S232 S233 S234 S235 S236 S237 S238 S239 S240 S241 S242 | S243 S244 S245 S246 S247 S248 S249 S250 | S251 S252 S253 S254 S255 S256 S257 S258 S259 S260 S261 S262 S263 S264 S265 | S266 S267 S268 S269 S270 S271 S272 S273 S274 S275 S276 S277 S278 | L0 L1 L2 L3 makes body 1
extrude "Extrude2" add sketch "Imported SVG" along normal blind 4 contours S0 S1 S2 S3 S4 S5 S6 S7 S8 S9 S10 S11 S12 S13 S14 S15 S16 S17 S18 S19 S20 S21 S22 S23 S24 S25 S26 S27 S28 S29 S30 S31 S32 S33 S34 S35 S36 S37 S38 S39 S40 S41 S42 S43 S44 S45 S46 S47 S48 S49 S50 S51 S52 | S201 S202 S203 S204 S205 S206 S207 S208 S209 S210 S211 S212 S213 S214 S215 S216 S217 | S218 S219 S220 S221 S222 S223 | S224 S225 S226 S227 S228 S229 bodies 1
box "BoxPrimitive1" add length 174.413 width 230.653 height 15 placed x (0, 1, 0) y (1, 0, 0) z (0, 0, -1) at (-110.6847, -91.5939, -5) separate body makes body 2
fillet "Fillet1" radius 50 tangency weight 2 8 edges at (-110.6847, -91.5939, -2.5) (-110.6847, 82.8194, -2.5) (119.968, 82.8194, -2.5) (119.968, -91.5939, -2.5) (-110.6847, -91.5939, -12.5) (-110.6847, 82.8191, -12.5) (119.9683, 82.8191, -12.5) (119.9683, -91.5939, -12.5) on bodies 1 2
chamfer "Chamfer1" distance 3 angle 45 8 edges at (4.6417, -91.5939, 0) (-100.4442, -81.1229, 0) (-110.6847, -4.3873, 0) (-100.2136, 72.5789, 0) (4.6417, 82.8194, 0) (109.7276, 72.3483, 0) (119.968, -4.3873, 0) (109.497, -81.3535, 0) on bodies 1
named bodies: "Stamp-TPU", "Backer-PLA"
